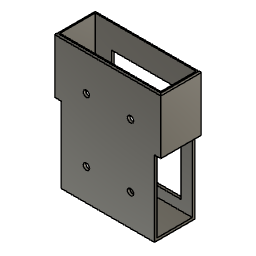
cuzorCase.v1 (Autodesk Fusion 360 design; units mm, degrees)
Autodesk Fusion 360 part; units mm, degrees
sketch "Sketch1" plane through (0, 0, 0) normal (0, 1, 0) x (1, 0, 0) in component "Case"
  line L0 (0, 0) -> (84, 0)
  line L1 (84, 0) -> (84, -104)
  line L2 (84, -104) -> (0, -104)
  line L3 (0, -104) -> (0, 0)
  dimension "d1" = 84
  dimension "d2" = 104
  constraint horizontal L0
  constraint vertical L1
  constraint horizontal L2
  constraint vertical L3
  constraint coincident L0.start L3.end
  measures "d1" distance of L0.start L0.end
  measures "d2" distance of L0.start L2.end
extrude "Extrude1" add sketch "Sketch1" along normal blind 32 in component "Case"
shell "Shell1" thickness 2 removed faces 1 at (56, 10.6667, 104) in component "Case"
fillet "Fillet1" radius 1 4 edges at (0, 16, 104) (42, 32, 104) (84, 16, 104) (42, 0, 104) in component "Case"
sketch "Sketch2" plane through (84, 0, 0) normal (1, 0, 0) x (0, 1, 0) in component "Case"
  line L0 (32, 103) -> (0, 103)
  line L1 (0, 103) -> (0, 0)
  line L2 (0, 0) -> (32, 0)
  line L3 (32, 0) -> (32, 103)
  line L4 (0, 0) -> (32, 0)
  line L5 (32, 0) -> (32, 60)
  line L6 (32, 60) -> (0, 60)
  line L7 (0, 60) -> (0, 0)
  dimension "d8" = 60
  constraint horizontal L4
  constraint vertical L5
  constraint horizontal L6
  constraint vertical L7
  constraint coincident L1.end L2.start
  measures "d8" distance of L1.end L6.end
extrude "Extrude2" cut sketch "Sketch2" against normal blind 5 contours L1 L2 L3 L4 L5 L6 L7 in component "Case"
sketch "Sketch3" plane through (0, 0, 0) normal (-1, 0, 0) x (0, -1, 0) in component "Case"
  line L0 (0, 103) -> (-32, 103)
  line L1 (-32, 103) -> (-32, 0)
  line L2 (-32, 0) -> (0, 0)
  line L3 (0, 0) -> (0, 103)
  line L4 (0, 0) -> (-32, 0)
  line L5 (-32, 0) -> (-32, 60)
  line L6 (-32, 60) -> (0, 60)
  line L7 (0, 60) -> (0, 0)
  dimension "d11" = 60
  constraint horizontal L4
  constraint vertical L5
  constraint horizontal L6
  constraint vertical L7
  constraint coincident L2.end L3.start
  measures "d11" distance of L2.end L6.end
extrude "Extrude3" cut sketch "Sketch3" against normal blind 5 contours L1 L2 L3 L4 L5 L6 L7 in component "Case"
sketch "Sketch4" plane through (0, 32, 0) normal (0, 1, 0) x (-1, 0, 0) in component "Case"
  line L0 (-5, 60) -> (0, 60)
  line L1 (0, 60) -> (0, 103)
  line L2 (0, 103) -> (-84, 103)
  line L3 (-84, 103) -> (-84, 60)
  line L4 (-84, 60) -> (-79, 60)
  line L5 (-79, 60) -> (-79, 0)
  line L6 (-79, 0) -> (-5, 0)
  line L7 (-5, 0) -> (-5, 60)
  line L8 (-70, 85) -> (-15, 85)
  line L9 (-15, 85) -> (-15, 10)
  line L10 (-15, 10) -> (-70, 10)
  line L11 (-70, 10) -> (-70, 85)
  line L12 (-70, 85) -> (-15, 85)
  line L13 (-15, 85) -> (-15, 10)
  line L14 (-15, 10) -> (-70, 10)
  line L15 (-70, 10) -> (-70, 85)
  constraint horizontal L8
  constraint vertical L9
  constraint horizontal L10
  constraint vertical L11
  constraint horizontal L12
  constraint vertical L13
  constraint horizontal L14
  constraint vertical L15
extrude "Extrude4" cut sketch "Sketch4" against normal blind 5 contours L8 L9 L10 L11 L12 L13 L14 L15 in component "Case"
sketch "Sketch5" plane through (0, 0, 0) normal (0, -1, 0) x (1, 0, 0) in component "Case"
  line L0 (0, 60) -> (5, 60)
  line L1 (5, 60) -> (5, 0)
  line L2 (5, 0) -> (79, 0)
  line L3 (79, 0) -> (79, 60)
  line L4 (79, 60) -> (84, 60)
  line L5 (84, 60) -> (84, 103)
  line L6 (84, 103) -> (0, 103)
  line L7 (0, 103) -> (0, 60)
  circle A0 centre (25, 75) radius 2.5
  circle A1 centre (60, 75) radius 2.5
  dimension "d16" = 5
  dimension "d17" = 5
  measures "d16" diameter of A0
  measures "d17" diameter of A1
extrude "Extrude5" cut sketch "Sketch5" against normal blind 5 contours A0 | A1 in component "Case"
sketch "Sketch6" plane through (0, 0, 0) normal (0, -1, 0) x (1, 0, 0) in component "Case"
  circle A0 centre (25, 75) radius 2.5
  circle A1 centre (60, 75) radius 2.5
  line L0 (0, 60) -> (5, 60)
  line L1 (5, 60) -> (5, 0)
  line L2 (5, 0) -> (79, 0)
  line L3 (79, 0) -> (79, 60)
  line L4 (79, 60) -> (84, 60)
  line L5 (84, 60) -> (84, 103)
  line L6 (84, 103) -> (0, 103)
  line L7 (0, 103) -> (0, 60)
  circle A2 centre (25, 25) radius 2.5
  circle A3 centre (60, 25) radius 2.5
extrude "Extrude6" cut sketch "Sketch6" against normal blind 5 contours A2 | A3 in component "Case"
component "Case" placed x (1, 0, 0) y (0, 1, 0) z (0, 0, 1) at (0, 0, 0)
